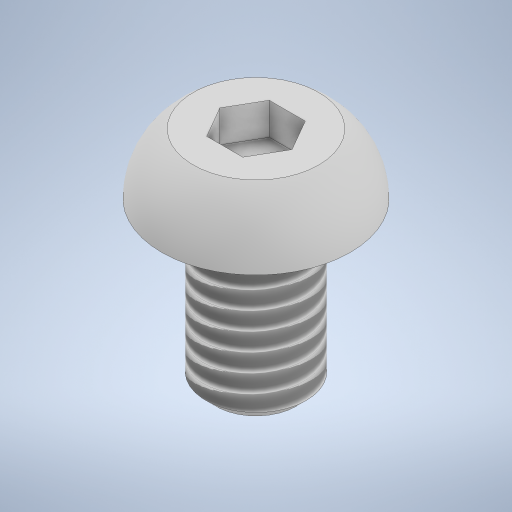
# Autodesk Inventor part: Vite ISO 7380
Saved by Autodesk Inventor 2023 (Build 270158000, 158)
## iProperties
Created: 2026-01-13
Part Number: Vite ISO 7380
Material: Generico
Document SubType Name: Modeling
Designer: Davide
Density: 1 g/cm^3
Appearance: Default
1_Materiale: − − −
2_Trattamento: − − −
3_Disegnato: D. Mitidieri
4_Controllato: C. Pirrottina
5_Approvato: S. Musella
Author: Davide
Autodesk Inventor part; units mm, degrees
ref_plane "YZ Plane" through (0, 0, 0) normal (1, 0, 0) x (0, 1, 0)
ref_plane "XZ Plane" through (0, 0, 0) normal (0, 1, 0) x (-1, 0, 0)
ref_plane "XY Plane" through (0, 0, 0) normal (0, 0, 1) x (1, 0, 0)
sketch "Schizzo2" plane through (0, 0, 0) normal (0, 0, 1) x (1, 0, 0)
  line L0 (0, 0) -> (0, 1.5)
  line L1 (0, 1.5) -> (1.5667, 1.5)
  line L2 (0, 0) -> (2.35, 0)
  arc A0 (2.35, 0) -> (1.5667, 1.5) centre (0.5222, 0) ccw
  dimension "d0" = 2.35
  dimension "d1" = 1.5
  dimension "d2" = 1.5667
  constraints: 6 end point, 2 point on circle, 1 centre point, 1 horizontal, 1 perpendicular, 1 point on line, 1 vertical
  measures "d0" distance from line of L0 L2.end
  measures "d1" distance between parallel lines of L2 L1
  measures "d2" distance from line of L0 L1.end
revolve "Rivoluzione1" add sketch "Schizzo2" angle 360 about axis through (0, 0, 0) along (0, 1, 0)
sketch "Schizzo3" plane through (0, 0, 0) normal (0, -1, 0) x (1, 0, 0)
  circle A0 centre (0, 0) radius 1.5667 projected
  circle A1 centre (0, 0) radius 1.25
  dimension "d4" = 2.5
  constraints: 1 centre point, 1 coincident
  measures "d4" diameter of A1
extrude "Estrusione1" add sketch "Schizzo3" along normal blind 4 contours A1
thread "Filettatura1" size "M2.5x0.45" class "6g" standard "ISO Metric profile" length 20
chamfer "Smusso1" distance 0.25 angle 45 1 edges at (-1.25, -4, 0) measured on face at (-0.1478, -4, -0.3896)
sketch "Schizzo4" plane through (0, 1.5, 0) normal (0, 1, 0) x (1, 0, 0)
  circle A0 centre (0, 0) radius 1.25 projected
  line L0 (0.4503, 0.78) -> (0.9007, 0)
  line L1 (0.9007, 0) -> (0.4503, -0.78)
  line L2 (0.4503, -0.78) -> (-0.4503, -0.78)
  line L3 (-0.4503, -0.78) -> (-0.9007, 0)
  line L4 (-0.9007, 0) -> (-0.4503, 0.78)
  line L5 (-0.4503, 0.78) -> (0.4503, 0.78)
  dimension "d12" = 1.56
  constraints: 12 end point, 1 coincident, 1 horizontal, 13 other
  measures "d12" distance between parallel lines of L2 L5
extrude "Estrusione2" cut sketch "Schizzo4" against normal blind 0.8 contours L0 L1 L2 L3 L4 L5
equation "\"d0\" = 0.5 * dk"
equation "\"d1\" = k"
equation "\"d2\" = 0.333333 * dk"
equation "\"d4\" = d"
equation "\"d5\" = L"
equation "\"d12\" = es"
equation "\"d13\" = t"
equation "\"t\" = 0.8"
equation "\"k\" = 1.5"
equation "\"d\" = 2.5"
equation "\"dk\" = 4.7"
equation "\"es\" = 1.56"
equation "\"L\" = 4"
